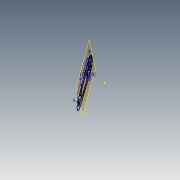
# Autodesk Inventor part: Upper ArmV
Saved by Autodesk Inventor 2014 SP1 (Build 180222100, 222)
## iProperties
Created: 2014-04-09
Part Number: Upper ArmV
Material: Generic
Document SubType Name: Modeling
Designer: tom
Density: 1 g/cm^3
Appearance: Default
Author: tom
Autodesk Inventor part; units mm, degrees
ref_plane "YZ Plane" through (0, 0, 0) normal (1, 0, 0) x (0, 1, 0)
ref_plane "XZ Plane" through (0, 0, 0) normal (0, 1, 0) x (-1, 0, 0)
ref_plane "XY Plane" through (0, 0, 0) normal (0, 0, 1) x (1, 0, 0)
ref_plane "Work Plane3" through (153.1742, 56.2271, -25.3358) normal (0.866, 0, -0.5) x (0.2088, 0.9086, 0.3617)
sketch "Sketch1" plane through (153.1742, 56.2271, -25.3358) normal (0.866, 0, -0.5) x (0.2088, 0.9086, 0.3617)
  circle A0 centre (0, 40) radius 3.175
  circle A1 centre (0, 0) radius 4.5
  circle A2 centre (0, 7.35) radius 0.65
  circle A3 centre (3.55, 7.35) radius 0.65
  circle A4 centre (-3.55, 7.35) radius 0.65
  line L0 (-7.1571, 40.5067) -> (-9.975, 0.7063)
  line L1 (7.1571, 40.5067) -> (9.975, 0.7062)
  line L2 (-3.8097, 31.1475) -> (-5.186, 11.7092)
  line L3 (3.8097, 31.1475) -> (5.186, 11.7092)
  arc A5 (-1.4191, 32.9667) -> (1.4191, 32.9667) centre (0, 40) ccw
  arc A6 (7.1571, 40.5067) -> (-7.1571, 40.5067) centre (0, 40) ccw
  arc A7 (-9.975, 0.7063) -> (9.975, 0.7062) centre (0, 0) ccw
  arc A8 (2.6592, 9.64) -> (-2.6591, 9.64) centre (0, 0) ccw
  arc A9 (-5.186, 11.7092) -> (-2.6591, 9.64) centre (-3.191, 11.568) ccw
  arc A10 (2.6592, 9.64) -> (5.186, 11.7092) centre (3.191, 11.568) ccw
  arc A11 (-1.4191, 32.9667) -> (-3.8097, 31.1475) centre (-1.8147, 31.0063) ccw
  arc A12 (3.8097, 31.1475) -> (1.4191, 32.9667) centre (1.8147, 31.0063) ccw
  circle A13 centre (-7.35, 0) radius 0.65
  circle A14 centre (-7.35, 3.55) radius 0.65
  circle A15 centre (-7.35, -3.55) radius 0.65
  circle A16 centre (0, -7.35) radius 0.65
  circle A17 centre (-3.55, -7.35) radius 0.65
  circle A18 centre (3.55, -7.35) radius 0.65
  circle A19 centre (7.35, 0) radius 0.65
  circle A20 centre (7.35, -3.55) radius 0.65
  circle A21 centre (7.35, 3.55) radius 0.65
  point P0 (-73.9118, -26.1665)
  point P1 (-3.6215, 33.806)
  point P2 (-5.42, 8.4038)
  point P3 (3.6215, 33.806)
  point P4 (5.42, 8.4038)
  dimension "d0" = 40
  dimension "d1" = 9
  dimension "d2" = 1.3
  dimension "d3" = 7.35
  dimension "d4" = 1.3
  dimension "d5" = 1.3
  dimension "d6" = 6.35
  dimension "d8" = 4
  dimension "d9" = 4
  dimension "d10" = 2
  dimension "d13" = 360
  constraints: 22 centre point, 20 point on circle, 12 tangent, 8 end point, 4 point on line, 3 equal radius, 25 other
  measures "d0" distance of A1.centre A0.centre
  measures "d1" diameter of A1
  measures "d2" diameter of A2
  measures "d3" distance of A1.centre A2.centre
  measures "d4" diameter of A3
  measures "d5" diameter of A4
  measures "d6" diameter of A0
  measures "d8" distance between parallel lines of L2 L0
  measures "d9" distance between parallel lines of L1 L3
  measures "d10" radius of A9
extrude "Extrusion1" add sketch "Sketch1" along normal blind 5.66
body "Solid1"
